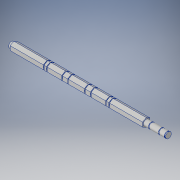
# Autodesk Inventor part: Flywheel Axle
Saved by Autodesk Inventor 2019.4 (Build 234330000, 330)
## iProperties
Created: 2020-01-18
Part Number: Flywheel Axle
Material: Aluminum 6061
Document SubType Name: Modeling
Designer: admin
Density: 2.7 g/cm^3
Appearance: Aluminum - Flat
Mass: 91.5408 g
Surface Area: 120.082 cm^2
Volume: 33.904 cm^3
Author: admin
Autodesk Inventor part; units mm, degrees
ref_plane "YZ Plane" through (0, 0, 0) normal (1, 0, 0) x (0, 1, 0)
ref_plane "XZ Plane" through (0, 0, 0) normal (0, 1, 0) x (-1, 0, 0)
ref_plane "XY Plane" through (0, 0, 0) normal (0, 0, 1) x (1, 0, 0)
sketch "Sketch1" plane through (0, 0, 0) normal (0, 0, 1) x (1, 0, 0)
  line L0 (0, 0) -> (0, 5)
  line L1 (0, 5) -> (4, 5)
  line L2 (4, 5) -> (4, 8.89)
  line L3 (4, 8.89) -> (230.2, 8.89)
  line L4 (230.2, 8.89) -> (230.2, 5)
  line L5 (268.1, 5) -> (268.1, 0)
  line L6 (268.1, 0) -> (0, 0)
  line L7 (230.2, 5) -> (238.8, 5)
  line L8 (238.8, 5) -> (238.8, 4.65)
  line L9 (238.8, 4.65) -> (239.9, 4.65)
  line L10 (239.9, 4.65) -> (239.9, 5)
  line L11 (239.9, 5) -> (255.9, 5)
  line L12 (255.9, 5) -> (255.9, 4.65)
  line L13 (255.9, 4.65) -> (257, 4.65)
  line L14 (257, 4.65) -> (257, 5)
  line L15 (257, 5) -> (265.9, 5)
  line L16 (265.9, 5) -> (265.9, 4.75)
  line L17 (265.9, 4.75) -> (267, 4.75)
  line L18 (267, 4.75) -> (267, 5)
  line L19 (267, 5) -> (268.1, 5)
  dimension "d0" = 226.2
  dimension "d1" = 5
  dimension "d2" = 8.89
  dimension "d3" = 4
  dimension "d4" = 1.1
  dimension "d5" = 0.35
  dimension "d6" = 1.1
  dimension "d7" = 8.6
  dimension "d8" = 16
  dimension "d9" = 1.1
  dimension "d10" = 0.25
  dimension "d11" = 26
  dimension "d12" = 1.1
  constraints: 40 end point, 14 perpendicular, 8 point on line, 2 horizontal, 1 vertical
  measures "d0" distance of L2.end L3.end
  measures "d1" distance between parallel lines of L6 L1
  measures "d2" distance between parallel lines of L6 L3
  measures "d3" distance of L0.end L1.end
  measures "d4" distance of L8.end L9.end
  measures "d5" distance of L7.end L8.end
  measures "d6" distance of L12.end L13.end
  measures "d7" distance between parallel lines of L4 L8
  measures "d8" distance of L10.end L11.end
  measures "d9" distance of L16.end L17.end
  measures "d10" distance of L15.end L16.end
  measures "d11" distance between parallel lines of L16 L10
  measures "d12" distance of L18.end L5.start
revolve "Revolution1" add sketch "Sketch1" angle 360 about axis through (268.1, 0, 0) along (-1, 0, 0)
sketch "Sketch2" plane through (230.2, 0, 0) normal (1, 0, 0) x (0, 0, -1)
  circle A0 centre (0, 0) radius 5 projected
  circle A1 centre (0, 0) radius 8.89 projected
  line L0 (0, 7.259) -> (6.2865, 3.6295)
  line L1 (6.2865, 3.6295) -> (6.2865, -3.6295)
  line L2 (6.2865, -3.6295) -> (0, -7.259)
  line L3 (0, -7.259) -> (-6.2865, -3.6295)
  line L4 (-6.2865, -3.6295) -> (-6.2865, 3.6295)
  line L5 (-6.2865, 3.6295) -> (0, 7.259)
  dimension "d14" = 12.573
  constraints: 12 end point, 1 coincident, 1 vertical, 13 other
  measures "d14" distance between parallel lines of L4 L1
extrude "Extrusion1" cut sketch "Sketch2" against normal through all contours A1
ref_plane "Work Plane1" through (167.1, -3.6295, 6.2865) normal (1, 0, 0) x (0, 0, -1)
sketch "Sketch3" plane through (167.1, -3.6295, 6.2865) normal (1, 0, 0) x (0, 0, -1)
  circle A0 centre (6.2865, 3.6295) radius 5.65
  line L0 (0, 7.259) -> (6.2865, 10.8885) projected
  line L1 (6.2865, 10.8885) -> (12.573, 7.259) projected
  line L2 (12.573, 7.259) -> (12.573, 0) projected
  line L3 (12.573, 0) -> (6.2865, -3.6295) projected
  line L4 (6.2865, -3.6295) -> (0, 0) projected
  line L5 (0, 0) -> (0, 7.259) projected
  circle A1 centre (6.2865, 3.6295) radius 5 construction
  dimension "d18" = 11.3
  constraints: 1 centre point, 1 coincident
  measures "d18" diameter of A0
extrude "Extrusion2" cut sketch "Sketch3" along normal blind 1.1
ref_plane "Work Plane2" through (142.1, -3.6295, 6.2865) normal (1, 0, 0) x (0, 0, -1)
sketch "Sketch4" plane through (142.1, -3.6295, 6.2865) normal (1, 0, 0) x (0, 0, -1)
  circle A0 centre (6.2865, 3.6295) radius 5.65 projected
  line L0 (6.2865, 10.8885) -> (0, 7.259) projected
  line L1 (12.573, 7.259) -> (6.2865, 10.8885) projected
  line L2 (12.573, 0) -> (12.573, 7.259) projected
  line L3 (6.2865, -3.6295) -> (12.573, 0) projected
  line L4 (0, 0) -> (6.2865, -3.6295) projected
  line L5 (0, 7.259) -> (0, 0) projected
extrude "Extrusion3" cut sketch "Sketch4" against normal blind 1.1
ref_plane "Work Plane3" through (117.1, -3.6295, 6.2865) normal (1, 0, 0) x (0, 0, -1)
mirror "Mirror1" about plane through (117.1, -3.6295, 6.2865) normal (1, 0, 0) of "Extrusion3", "Extrusion2"
ref_plane "Work Plane4" through (103.3, -3.6295, -6.2865) normal (-1, 0, 0) x (0, 0, 1)
sketch "Sketch5" plane through (103.3, -3.6295, -6.2865) normal (-1, 0, 0) x (0, 0, 1)
  circle A0 centre (6.2865, 3.6295) radius 5.65 projected
  line L0 (12.573, 7.259) -> (6.2865, 10.8885) projected
  line L1 (12.573, 0) -> (12.573, 7.259) projected
  line L2 (6.2865, -3.6295) -> (12.573, 0) projected
  line L3 (0, 0) -> (6.2865, -3.6295) projected
  line L4 (0, 7.259) -> (0, 0) projected
  line L5 (6.2865, 10.8885) -> (0, 7.259) projected
extrude "Extrusion4" cut sketch "Sketch5" along normal blind 1.1
ref_plane "Work Plane5" through (61.752, -3.6295, -6.2865) normal (-1, 0, 0) x (0, 0, 1)
sketch "Sketch6" plane through (61.752, -3.6295, -6.2865) normal (-1, 0, 0) x (0, 0, 1)
  circle A0 centre (6.2865, 3.6295) radius 5.65 projected
  line L0 (6.2865, 10.8885) -> (12.573, 7.259) projected
  line L1 (0, 7.259) -> (6.2865, 10.8885) projected
  line L2 (0, 0) -> (0, 7.259) projected
  line L3 (6.2865, -3.6295) -> (0, 0) projected
  line L4 (12.573, 0) -> (6.2865, -3.6295) projected
  line L5 (12.573, 7.259) -> (12.573, 0) projected
extrude "Extrusion5" cut sketch "Sketch6" along normal blind 1.1
mirror "Mirror2" about plane through (117.1, -3.6295, 6.2865) normal (1, 0, 0) of "Extrusion4", "Extrusion5"
body "Solid1"
